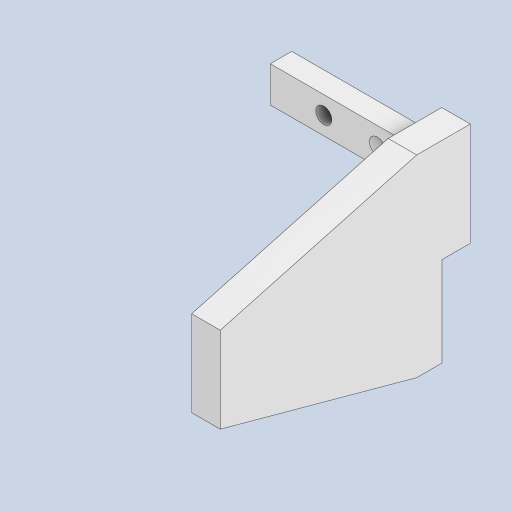
# Autodesk Inventor part: left-nail
Saved by Autodesk Inventor 2023 (Build 270158000, 158)
## iProperties
Created: 2024-11-28
Part Number: left-nail
Material: ABS プラスチック
Document SubType Name: Modeling
Designer: kiyo
Density: 1.06 g/cm^3
Appearance: 滑らか - 白
Author: kiyo
Autodesk Inventor part; units mm, degrees
ref_plane "YZ Plane" through (0, 0, 0) normal (1, 0, 0) x (0, 1, 0)
ref_plane "XZ Plane" through (0, 0, 0) normal (0, 1, 0) x (-1, 0, 0)
ref_plane "XY Plane" through (0, 0, 0) normal (0, 0, 1) x (1, 0, 0)
sketch "スケッチ2" plane through (0, 0, 0) normal (1, 0, 0) x (0, 1, 0)
  line L0 (-50, 46.625) -> (0, 46.625)
  line L1 (0, 46.625) -> (0, 36.625)
  line L2 (0, 36.625) -> (-50, 36.625)
  line L3 (-50, 36.625) -> (-50, 46.625)
  line L4 (0, 36.625) -> (-8, 36.625)
  line L5 (-8, 36.625) -> (-8, 0)
  line L6 (-8, 0) -> (0, 0)
  line L7 (0, 0) -> (0, 36.625)
  circle A0 centre (-20, 41.625) radius 2.25
  circle A1 centre (-35, 41.625) radius 2.25
  line L8 (-8, 36.625) -> (0, 36.625)
  line L9 (0, 36.625) -> (0, 54)
  line L10 (0, 54) -> (-8, 54)
  line L11 (-8, 54) -> (-8, 36.625)
  point P0 (-8, 46.625)
  point P1 (0, 46.625)
  dimension "d7" = 50
  dimension "d8" = 10
  dimension "d10" = 8
  dimension "d11" = 4.5
  dimension "d12" = 4.5
  dimension "d13" = 15
  dimension "d14" = 20
  dimension "d15" = 5
  dimension "d16" = 5
  dimension "d27" = 54
  dimension "d28" = 7.375
  constraints: 24 end point, 6 parallel, 3 horizontal, 3 perpendicular, 2 centre point, 1 coincident, 1 collinear
  measures "d7" distance of L0.start L0.end
  measures "d8" distance between parallel lines of L2 L0
  measures "d10" distance of L5.end L6.end
  measures "d11" diameter of A0
  measures "d12" diameter of A1
  measures "d13" distance of A0.centre A1.centre
  measures "d14" distance from line of L1 A0.centre
  measures "d15" distance from line of L0 A0.centre
  measures "d16" distance from line of L0 A1.centre
  measures "d27" distance between parallel lines of L6 L10
  measures "d28" distance between parallel lines of L0 L10
extrude "押し出し2" add sketch "スケッチ2" along normal blind 6 contours L0 L11 L2 L3
extrude "押し出し5" add sketch "スケッチ2" along normal blind 70 contours L11 L10 L9 L0 | L0 L1 L2 L11 | L2 L7 L6 L5
sketch "スケッチ4" plane through (0, -8, 0) normal (0, -1, 0) x (1, 0, 0)
  line L0 (70, 0) -> (70, 54) projected
  line L1 (70, 15) -> (15, 0)
  line L2 (15, 0) -> (15, 54)
  line L3 (15, 54) -> (70, 39)
  line L4 (0, 54) -> (70, 54) projected
  line L5 (0, 36.625) -> (0, 0) projected
  line L6 (0, 0) -> (70, 0) projected
  line L7 (0, 25.077) -> (7.9173, 25.077)
  line L8 (7.9173, 25.077) -> (7.9173, 0)
  line L9 (7.9173, 0) -> (0, 0)
  line L10 (0, 0) -> (0, 25.077)
  dimension "d31" = 15
  dimension "d32" = 15
  dimension "d33" = 15
  constraints: 14 end point, 6 point on line, 3 parallel, 1 horizontal, 1 perpendicular
  measures "d31" distance from line of L3.end L4
  measures "d32" distance of L0.start L1.start
  measures "d33" distance between parallel lines of L5 L2
extrude "押し出し6" cut sketch "スケッチ4" against normal blind 8 contours L6 L1 L0 | L6 L5 L7 L8 | L3 L4 L0
sketch "スケッチ5" plane through (0, 0, 54) normal (0, 1, 0) x (1, 0, 0)
  line L0 (15, 0) -> (70, 15) projected
  line L1 (70, 39) -> (15, 54) projected
  line L2 (70.01, 38.9973) -> (70.01, 15.0027)
  line L3 (70, 15) -> (15, 0) projected
  line L4 (70, 39) -> (70, 15) projected
  line L5 (70.01, 15.0027) -> (70, 15)
  line L6 (70.01, 38.9973) -> (70, 39)
  point P0 (0, 54)
  dimension "d37" = 0.01
  constraints: 6 end point, 2 point on line, 1 vertical
  measures "d37" distance between parallel lines of L4 L2
extrude "押し出し7" add sketch "スケッチ5" against normal blind 8
